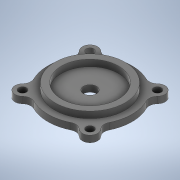
# Autodesk Inventor part: Lid
Saved by Autodesk Inventor 2020.2 (Build 242310000, 310)
## iProperties
Created: 2020-09-02
Part Number: Lid
Material: Generic
Document SubType Name: Modeling
Designer: JK
Density: 1 g/cm^3
Appearance: Smooth - Black
Author: JK
Autodesk Inventor part; units mm, degrees
ref_plane "YZ Plane" through (0, 0, 0) normal (1, 0, 0) x (0, 1, 0)
ref_plane "XZ Plane" through (0, 0, 0) normal (0, 1, 0) x (-1, 0, 0)
ref_plane "XY Plane" through (0, 0, 0) normal (0, 0, 1) x (1, 0, 0)
sketch "Sketch1" plane through (0, 0, 0) normal (0, 1, 0) x (-1, 0, 0)
  line L0 (-21, 21) -> (21, 21)
  line L1 (21, 21) -> (21, -21)
  line L2 (21, -21) -> (-21, -21)
  line L3 (-21, -21) -> (-21, 21)
  line L4 (-21, 21) -> (21, -21) construction
  line L5 (21, 21) -> (-21, -21) construction
  point P0 (0, 0)
  dimension "d0" = 42
  dimension "d1" = 42
  constraints: 12 end point, 2 midpoint, 2 parallel, 1 horizontal, 1 perpendicular
  measures "d0" distance of L0.end L1.end
  measures "d1" distance of L1.end L2.end
extrude "Extrusion1" add sketch "Sketch1" along normal blind 3
sketch "Sketch2" plane through (0, 3, 0) normal (0, 1, 0) x (1, 0, 0)
  circle A0 centre (0, 0) radius 3
  circle A1 centre (-15.5, -15.5) radius 1.8
  circle A2 centre (-15.5, 15.5) radius 1.8
  circle A3 centre (15.5, 15.5) radius 1.8
  circle A4 centre (15.5, -15.5) radius 1.8
  dimension "d4" = 6
  dimension "d5" = 3.6
  dimension "d6" = 31
  dimension "d7" = 15.5
  dimension "d8" = 15.5
  dimension "d9" = 31
  constraints: 5 centre point, 3 equal radius, 2 horizontal alignment, 2 vertical alignment, 1 coincident
  measures "d4" diameter of A0
  measures "d5" diameter of A1
  measures "d6" distance of A2.centre A1.centre
  measures "d7" horizontal distance of A1.centre point (0, 0)
  measures "d8" horizontal distance of A1.centre point (0, 0)
  measures "d9" distance of A4.centre A1.centre
extrude "Extrusion2" cut sketch "Sketch2" against normal blind 10
sketch "Sketch3" plane through (0, 3, 0) normal (0, 1, 0) x (1, 0, 0)
  circle A0 centre (-15.5, -15.5) radius 1.8 projected
  circle A1 centre (-15.5, -15.5) radius 3.5
  circle A2 centre (0, 0) radius 19.3
  line L0 (-13.0251, -17.9749) -> (-10.946, -15.8958)
  line L1 (-17.9749, -13.0251) -> (-15.8958, -10.946)
  circle A3 centre (15.5, -15.5) radius 1.8 projected
  circle A4 centre (15.5, -15.5) radius 3.5
  circle A5 centre (15.5, 15.5) radius 1.8 projected
  circle A6 centre (15.5, 15.5) radius 3.5
  circle A7 centre (-15.5, 15.5) radius 1.8 projected
  circle A8 centre (-15.5, 15.5) radius 3.5
  line L2 (13.0251, -17.9749) -> (10.946, -15.8958)
  line L3 (17.9749, -13.0251) -> (15.8958, -10.946)
  line L4 (13.0251, 17.9749) -> (10.946, 15.8958)
  line L5 (17.9749, 13.0251) -> (15.8958, 10.946)
  line L6 (-15.8958, 10.946) -> (-17.9749, 13.0251)
  line L7 (-10.946, 15.8958) -> (-13.0251, 17.9749)
  circle A9 centre (15.5, 15.5) radius 1.8 projected
  circle A10 centre (-15.5, 15.5) radius 1.8 projected
  circle A11 centre (15.5, -15.5) radius 1.8 projected
  circle A12 centre (-15.5, -15.5) radius 1.8 projected
  circle A13 centre (0, 0) radius 3 projected
  line L8 (-21, 21) -> (-21, -21) projected
  line L9 (-21, -21) -> (21, -21) projected
  line L10 (21, -21) -> (21, 21) projected
  line L11 (21, 21) -> (-21, 21) projected
  dimension "d13" = 38.6
  dimension "d12" = 7
  constraints: 16 end point, 8 point on circle, 8 tangent, 6 parallel, 5 coincident, 4 centre point, 3 equal radius, 1 perpendicular, 1 point on line, 10 other
  measures "d12" diameter of A1
extrude "Extrusion3" cut sketch "Sketch3" against normal blind 10 contours L11 L10 L9 L8
sketch "Sketch4" plane through (0, 3, 0) normal (0, 1, 0) x (1, 0, 0)
  circle A0 centre (0, 0) radius 3 projected
  circle A1 centre (0, 0) radius 16.125
  circle A2 centre (0, 0) radius 13.125
  dimension "d16" = 32.25
  dimension "d17" = 3
  constraints: 2 centre point, 2 coincident
  measures "d16" diameter of A1
  measures "d17" radial gap between concentric circles of A1 A2
extrude "Extrusion4" add sketch "Sketch4" along normal blind 3 contours A1
fillet "Fillet1" radius 4 8 edges at (-15.8958, 1.5, -10.946) (-15.8958, 1.5, 10.946) (-10.946, 1.5, 15.8958) (10.946, 1.5, 15.8958) (15.8958, 1.5, 10.946) (15.8958, 1.5, -10.946) (10.946, 1.5, -15.8958) (-10.946, 1.5, -15.8958)
body "Solid1"
